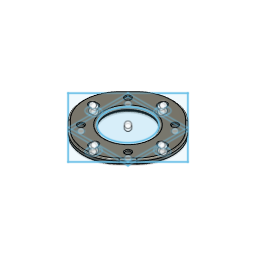
Component34 (Autodesk Fusion 360 design; units mm, degrees)
Autodesk Fusion 360 part; units mm, degrees
sketch "sketch 1634" plane through (0, 29.0232, 0) normal (0, 1, 0) x (-1, 0, 0)
  circle A0 centre (-113.2386, -613.9849) radius 1.6
  circle A1 centre (-83.2386, -613.9849) radius 1.6
  circle A2 centre (-113.2386, -583.9849) radius 1.6
  circle A3 centre (-83.2386, -583.9849) radius 1.6
  line L0 (-79.2386, -617.9849) -> (-79.2386, -579.9849)
  line L1 (-79.2386, -579.9849) -> (-117.2386, -579.9849)
  line L2 (-117.2386, -579.9849) -> (-117.2386, -617.9849)
  line L3 (-117.2386, -617.9849) -> (-79.2386, -617.9849)
extrude "Extrude1" add sketch "sketch 1634" along normal blind 2
sketch "sketch 1668" plane through (0.1033, 31.0232, 0) normal (0, 1, 0) x (-1, 0, 0)
  line L0 (-79.1352, -617.9849) -> (-60.0433, -598.893)
  line L1 (-60.0433, -598.893) -> (-98.0433, -560.893)
  line L2 (-98.0433, -560.893) -> (-117.1352, -579.9849)
  line L3 (-79.1352, -579.9849) -> (-117.1352, -579.9849)
  line L4 (-79.1352, -617.9849) -> (-79.1352, -579.9849)
  line L5 (-117.1352, -579.9849) -> (-136.2271, -599.0768)
  line L6 (-136.2271, -599.0768) -> (-98.2271, -637.0768)
  line L7 (-98.2271, -637.0768) -> (-79.1352, -617.9849)
  line L8 (-117.1352, -617.9849) -> (-79.1352, -617.9849)
  line L9 (-117.1352, -579.9849) -> (-117.1352, -617.9849)
extrude "Extrude2" add sketch "sketch 1668" against normal blind 2 contours L0 L1 L2 L3 L4 | L5 L6 L7 L8 L9
sketch "sketch 1704" plane through (-79.8299, 31.0232, -43.2833) normal (0, 1, 0) x (-1, 0, 0)
  circle A0 centre (-178.0685, -555.7015) radius 1
extrude "Extrude3" cut sketch "sketch 1704" against normal blind 6.5
sketch "sketch 1716" plane through (-79.8299, 32.0232, -43.2833) normal (0, 1, 0) x (-1, 0, 0)
  arc A0 (-176.2685, -533.0741) -> (-179.8685, -533.0741) centre (-178.0685, -533.0741) ccw
  line L0 (-179.8685, -534.4883) -> (-179.8685, -533.0741)
  arc A1 (-179.8685, -534.4883) -> (-176.2685, -534.4883) centre (-178.0685, -534.4883) ccw
  line L1 (-176.2685, -533.0741) -> (-176.2685, -534.4883)
  arc A2 (-156.8553, -553.9015) -> (-156.8553, -557.5015) centre (-156.8553, -555.7015) ccw
  line L2 (-155.441, -557.5015) -> (-156.8553, -557.5015)
  arc A3 (-155.441, -557.5015) -> (-155.441, -553.9015) centre (-155.441, -555.7015) ccw
  line L3 (-156.8553, -553.9015) -> (-155.441, -553.9015)
  arc A4 (-176.2685, -576.9147) -> (-179.8685, -576.9147) centre (-178.0685, -576.9147) ccw
  line L4 (-179.8685, -578.3289) -> (-179.8685, -576.9147)
  arc A5 (-179.8685, -578.3289) -> (-176.2685, -578.3289) centre (-178.0685, -578.3289) ccw
  line L5 (-176.2685, -576.9147) -> (-176.2685, -578.3289)
  arc A6 (-200.6959, -553.9015) -> (-200.6959, -557.5015) centre (-200.6959, -555.7015) ccw
  line L6 (-199.2817, -557.5015) -> (-200.6959, -557.5015)
  arc A7 (-199.2817, -557.5015) -> (-199.2817, -553.9015) centre (-199.2817, -555.7015) ccw
  line L7 (-200.6959, -553.9015) -> (-199.2817, -553.9015)
extrude "Extrude4" cut sketch "sketch 1716" against normal blind 18
sketch "sketch 1792" plane through (-115.9515, 31.0232, -28.364) normal (0, 1, 0) x (-1, 0, 0)
  circle A0 centre (-214.19, -570.6209) radius 1
extrude "Extrude5" add sketch "sketch 1792" against normal blind 2
fillet "Fillet1" radius 23 4 edges at (136.3305, 30.0232, -599.0768) (98.1467, 30.0232, -560.893) (60.1467, 30.0232, -598.893) (98.3305, 30.0232, -637.0768)
extrude "Extrude6" add 1 faces at (98.1937, 31.0232, -592.6018) along direction (0, 1, 0) blind 2
extrude "Extrude7" cut 1 faces at (98.1937, 33.0232, -592.6018) along direction (0, -1, 0) blind 0.5
sketch "sketch 1804" plane through (148.0133, 29.0232, -134.823) normal (0, -1, 0) x (1, 0, 0)
  arc A0 (-47.9747, -442.9487) -> (-51.5747, -442.9487) centre (-49.7747, -442.9487) cw
  line L0 (-51.5747, -442.9487) -> (-51.5747, -441.5344)
  arc A1 (-51.5747, -441.5344) -> (-47.9747, -441.5344) centre (-49.7747, -441.5344) cw
  line L1 (-47.9747, -441.5344) -> (-47.9747, -442.9487)
  arc A2 (-53.1747, -442.9487) -> (-46.3747, -442.9487) centre (-49.7747, -442.9487) ccw
  line L2 (-46.3747, -441.5344) -> (-46.3747, -442.9487)
  arc A3 (-46.3747, -441.5344) -> (-53.1747, -441.5344) centre (-49.7747, -441.5344) ccw
  line L3 (-53.1747, -442.9487) -> (-53.1747, -441.5344)
  arc A4 (-47.9747, -486.7893) -> (-51.5747, -486.7893) centre (-49.7747, -486.7893) cw
  line L4 (-51.5747, -486.7893) -> (-51.5747, -485.3751)
  arc A5 (-51.5747, -485.3751) -> (-47.9747, -485.3751) centre (-49.7747, -485.3751) cw
  line L5 (-47.9747, -485.3751) -> (-47.9747, -486.7893)
  arc A6 (-46.3747, -485.3751) -> (-53.1747, -485.3751) centre (-49.7747, -485.3751) ccw
  line L6 (-53.1747, -486.7893) -> (-53.1747, -485.3751)
  arc A7 (-53.1747, -486.7893) -> (-46.3747, -486.7893) centre (-49.7747, -486.7893) ccw
  line L7 (-46.3747, -485.3751) -> (-46.3747, -486.7893)
  arc A8 (-28.5615, -465.9619) -> (-28.5615, -462.3619) centre (-28.5615, -464.1619) cw
  line L8 (-28.5615, -462.3619) -> (-27.1473, -462.3619)
  arc A9 (-27.1473, -462.3619) -> (-27.1473, -465.9619) centre (-27.1473, -464.1619) cw
  line L9 (-27.1473, -465.9619) -> (-28.5615, -465.9619)
  arc A10 (-27.1473, -467.5619) -> (-27.1473, -460.7619) centre (-27.1473, -464.1619) ccw
  line L10 (-28.5615, -460.7619) -> (-27.1473, -460.7619)
  arc A11 (-28.5615, -460.7619) -> (-28.5615, -467.5619) centre (-28.5615, -464.1619) ccw
  line L11 (-27.1473, -467.5619) -> (-28.5615, -467.5619)
  arc A12 (-72.4021, -465.9619) -> (-72.4021, -462.3619) centre (-72.4021, -464.1619) cw
  line L12 (-72.4021, -462.3619) -> (-70.9879, -462.3619)
  arc A13 (-70.9879, -462.3619) -> (-70.9879, -465.9619) centre (-70.9879, -464.1619) cw
  line L13 (-70.9879, -465.9619) -> (-72.4021, -465.9619)
  arc A14 (-70.9879, -467.5619) -> (-70.9879, -460.7619) centre (-70.9879, -464.1619) ccw
  line L14 (-72.4021, -460.7619) -> (-70.9879, -460.7619)
  arc A15 (-72.4021, -460.7619) -> (-72.4021, -467.5619) centre (-72.4021, -464.1619) ccw
  line L15 (-70.9879, -467.5619) -> (-72.4021, -467.5619)
extrude "Extrude8" cut sketch "sketch 1804" against normal blind 2.6
fillet "Fillet2" radius 1 20 edges at (116.0518, 29.0232, -598.9849) (120.1589, 29.0232, -595.5849) (124.266, 29.0232, -598.9849) (120.1589, 29.0232, -602.3849) (98.2386, 29.0232, -572.9575) (101.6386, 29.0232, -577.0646) (98.2386, 29.0232, -581.1717) (94.8386, 29.0232, -577.0646) (81.7468, 29.0232, -584.5635) (111.7468, 29.0232, -584.5635) (111.7468, 29.0232, -614.5635) (98.2386, 29.0232, -625.0123) (94.8386, 29.0232, -620.9052) (98.2386, 29.0232, -616.7981) (101.6386, 29.0232, -620.9052) (81.7468, 29.0232, -614.5635) (72.2112, 29.0232, -598.9849) (76.3183, 29.0232, -595.5849) (80.4254, 29.0232, -598.9849) (76.3183, 29.0232, -602.3849)
fillet "Fillet3" radius 0.45 20 edges at (98.2386, 32.5232, -618.3981) (100.0386, 32.5232, -620.9052) (98.2386, 32.5232, -623.4123) (96.4386, 32.5232, -620.9052) (81.7468, 32.5232, -613.4063) (78.8254, 32.5232, -598.9849) (76.3183, 32.5232, -600.7849) (73.8112, 32.5232, -598.9849) (76.3183, 32.5232, -597.1849) (81.7468, 32.5232, -583.4063) (98.2386, 32.5232, -574.5575) (100.0386, 32.5232, -577.0646) (98.2386, 32.5232, -579.5717) (96.4386, 32.5232, -577.0646) (111.7468, 32.5232, -583.4063) (122.666, 32.5232, -598.9849) (120.1589, 32.5232, -600.7849) (117.6518, 32.5232, -598.9849) (120.1589, 32.5232, -597.1849) (111.7468, 32.5232, -613.4063)
sketch "sketch 1944" plane through (148.0133, 32.5232, -134.823) normal (0, 1, 0) x (-1, 0, 0)
  circle A0 centre (49.7747, -464.1619) radius 14
extrude "Extrude9" cut sketch "sketch 1944" against normal blind 9
fillet "Fillet4" radius 1.5 2 edges at (111.2912, 32.5232, -593.9223) (111.2912, 29.0232, -604.0475)
fillet "Fillet5" radius 1 16 edges at (69.6736, 32.5232, -598.893) (79.2386, 32.5232, -617.9849) (98.3305, 32.5232, -627.5498) (117.3305, 32.5232, -618.0768) (126.8035, 32.5232, -599.0768) (117.2386, 32.5232, -579.9849) (98.1467, 32.5232, -570.4199) (79.1467, 32.5232, -579.893) (117.2386, 29.0232, -579.9849) (126.8035, 29.0232, -599.0768) (117.3305, 29.0232, -618.0768) (98.3305, 29.0232, -627.5498) (79.2386, 29.0232, -617.9849) (69.6736, 29.0232, -598.893) (79.1467, 29.0232, -579.893) (98.1467, 29.0232, -570.4199)
